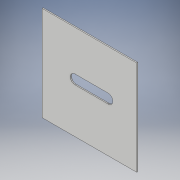
# Autodesk Inventor part: DecupajOvalizat1
Saved by Autodesk Inventor 2019 (Build 230136000, 136)
## iProperties
Created: 2020-04-08
Part Number: DecupajOvalizat1
Material: Generic
Document SubType Name: Sheet Metal
Designer: Gabriel
Density: 1 g/cm^3
Sheet Metal Rule: Default_mm
Appearance: Default
Author: Gabriel
Autodesk Inventor part; units mm, degrees
ref_plane "YZ Plane" through (0, 0, 0) normal (1, 0, 0) x (0, 1, 0)
ref_plane "XZ Plane" through (0, 0, 0) normal (0, 1, 0) x (-1, 0, 0)
ref_plane "XY Plane" through (0, 0, 0) normal (0, 0, 1) x (1, 0, 0)
sketch "Sketch1" plane through (0, 0, 0) normal (0, 0, 1) x (1, 0, 0)
  line L0 (-8.4106, 7.1523) -> (31.5894, 7.1523)
  line L1 (31.5894, 7.1523) -> (31.5894, -32.8477)
  line L2 (31.5894, -32.8477) -> (-8.4106, -32.8477)
  line L3 (-8.4106, -32.8477) -> (-8.4106, 7.1523)
  point P0 (0, 0)
  dimension "d0" = 40
  dimension "d1" = 40
  measures "d0" distance of L0.end L1.end
  measures "d1" distance of L1.end L2.end
extrude "Plate1" add sketch "Sketch1" along normal blind 0.5
sketch "Sketch2" plane through (0, 0, 0.5) normal (0, 0, 1) x (1, 0, 0)
  line L0 (19.5039, -11.896) -> (5.5039, -11.896) construction
  line L1 (19.5039, -9.896) -> (5.5039, -9.896)
  line L2 (5.5039, -13.896) -> (19.5039, -13.896)
  arc A0 (19.5039, -13.896) -> (19.5039, -9.896) centre (19.5039, -11.896) ccw
  arc A1 (5.5039, -9.896) -> (5.5039, -13.896) centre (5.5039, -11.896) ccw
  point P0 (0, 0)
  point P1 (12.5039, -11.896)
  dimension "LG_C" = 14
  dimension "LT_C" = 4
  constraints: 8 end point, 4 point on circle, 4 tangent, 2 centre point, 1 horizontal, 1 midpoint, 1 parallel
  measures "LG_C" distance of L0.start L0.end
  measures "LT_C" distance of L2.start L1.end
extrude "Cut1" cut sketch "Sketch2" against normal blind 0.5
equation "\"d5\" = Thickness"
equation "\"d2\" = Thickness"
equation "\"BendRadius\" = Thickness"
equation "\"BendReliefWidth\" = Thickness"
equation "\"BendReliefDepth\" = 0.5 * Thickness"
equation "\"CornerReliefSize\" = 4 * Thickness"
equation "\"MinimumRemnant\" = 2 * Thickness"
equation "\"TransitionRadius\" = BendRadius"
equation "\"JacobiRadiusSize\" = BendRadius"
equation "\"GapSize\" = Thickness"
equation "\"Thickness\" = 0.5"
body "Solid1"
